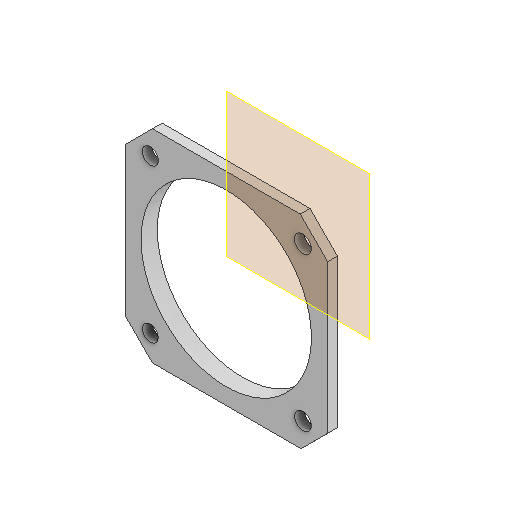
# Autodesk Inventor part: Pump_Lid
Saved by Autodesk Inventor 2022 (Build 260153000, 153)
## iProperties
Created: 2022-11-30
Part Number: Pump_Lid
Material: Generisch
Document SubType Name: Modeling
Designer: diederichbenedict
Density: 1 g/cm^3
Appearance: Vorgabe
Author: diederichbenedict
Autodesk Inventor part; units mm, degrees
ref_plane "YZ Plane" through (0, 0, 0) normal (1, 0, 0) x (0, 1, 0)
ref_plane "XZ Plane" through (0, 0, 0) normal (0, 1, 0) x (-1, 0, 0)
ref_plane "XY Plane" through (0, 0, 0) normal (0, 0, 1) x (1, 0, 0)
ref_plane "Arbeitsebene1" through (-58.716, -54.45, 1.8) normal (0, 0, 1) x (1, 0, 0)
sketch "Skizze1" plane through (-58.716, -54.45, 0) normal (0, 0, 1) x (1, 0, 0)
  circle A0 centre (-11.3643, -15.5584) radius 13.0833
  line L0 (4.216, -27.049) -> (4.216, -4.234)
  line L1 (4.216, -4.234) -> (0, 0)
  line L2 (0, 0) -> (-22.71, 0)
  line L3 (-22.71, 0) -> (-26.784, -4.092)
  line L4 (-26.784, -4.092) -> (-26.784, -27.049)
  line L5 (-26.784, -27.049) -> (-22.71, -31.14)
  line L6 (-22.71, -31.14) -> (0.142, -31.14)
  line L7 (0.142, -31.14) -> (4.216, -27.049)
  circle A1 centre (0.4286, -27.2971) radius 1.2941
  circle A2 centre (0.4173, -3.7431) radius 1.3039
  circle A3 centre (-23.0288, -3.7639) radius 1.2464
  circle A4 centre (-23.0166, -27.3387) radius 1.2172
  point P0 (58.716, 54.45)
  constraints: 16 end point, 5 centre point
extrude "Extrusion1" add sketch "Skizze1" along normal blind 1.5
sketch "Skizze2" plane through (-58.716, -54.45, 0) normal (0, 0, -1) x (-1, 0, 0)
  circle A0 centre (11.3643, -15.5584) radius 13.0833 projected
  circle A1 centre (11.3643, -15.5584) radius 14
  point P0 (-58.716, 54.45)
  dimension "d2" = 28
  constraints: 1 centre point, 1 coincident
  measures "d2" diameter of A1
extrude "Extrusion2" add sketch "Skizze2" along normal blind 1
